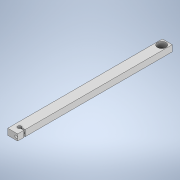
# Autodesk Inventor part: Arm
Saved by Autodesk Inventor 2021.3 (Build 253353000, 353)
## iProperties
Created: 2021-10-18
Part Number: Arm
Material: Generisch
Document SubType Name: Modeling
Designer: bhelg
Density: 1 g/cm^3
Appearance: Vorgabe
Author: bhelg
Autodesk Inventor part; units mm, degrees
ref_plane "YZ Plane" through (0, 0, 0) normal (1, 0, 0) x (0, 1, 0)
ref_plane "XZ Plane" through (0, 0, 0) normal (0, 1, 0) x (-1, 0, 0)
ref_plane "XY Plane" through (0, 0, 0) normal (0, 0, 1) x (1, 0, 0)
sketch "Skizze2" plane through (0, 0, 0) normal (0, 1, 0) x (-1, 0, 0)
  line L0 (0, 0) -> (16, 0)
  line L1 (16, 0) -> (16, 250)
  line L2 (16, 250) -> (0, 250)
  line L3 (0, 250) -> (0, 0)
  dimension "d0" = 16
  dimension "d1" = 250
  constraints: 8 end point, 2 parallel, 1 horizontal, 1 perpendicular
  measures "d0" distance of L2.end L1.end
  measures "d1" distance of L1.end L0.end
extrude "Extrusion1" add sketch "Skizze2" along normal blind 10
sketch "Skizze3" plane through (0, 0, 250) normal (1, 0, 0) x (0, 0, -1)
  line L0 (250, 0) -> (0, 0) projected
  line L1 (250, 10) -> (0, 10) projected
  line L2 (10, 0) -> (12, 0)
  line L3 (12, 0) -> (12, 10)
  line L4 (12, 10) -> (10, 10)
  line L5 (10, 10) -> (10, 0)
  line L6 (0, 0) -> (0, 10) projected
  point P0 (10, 10)
  point P1 (12, 0)
  dimension "d4" = 2
  dimension "d5" = 10
  constraints: 8 end point, 2 parallel, 2 point on line, 1 horizontal, 1 perpendicular
  measures "d4" distance between parallel lines of L3 L5
  measures "d5" distance between parallel lines of L6 L5
extrude "Extrusion2" cut sketch "Skizze3" against normal blind 7.5 contours L0 L5 L1 L3
sketch "Skizze4" plane through (-16, 0, 250) normal (0, 0, 1) x (1, 0, 0)
  line L0 (0, 0) -> (16, 0) projected
  line L1 (16, 0) -> (16, 10) projected
  point P0 (13.5, 5)
  dimension "d8" = 5
  dimension "d9" = 2.5
  measures "d8" distance from line of point (13.5, 5) L0
  measures "d9" distance from line of L1 point (13.5, 5)
hole "Bohrung1" at (-2.5, 5, 250) direction (0, 0, -1) diameter 4.2 depth 12
sketch "Skizze5" plane through (0, 10, 0) normal (0, 1, 0) x (1, 0, 0)
  line L0 (-16, -250) -> (0, -250) projected
  line L1 (-16, 0) -> (-16, -250) projected
  point P0 (0, 0)
  point P1 (-8, -239)
  dimension "d17" = 11
  dimension "d18" = 8
  measures "d17" distance from line of point (-8, -239) L0
  measures "d18" distance from line of L1 point (-8, -239)
hole "Bohrung2" at (-8, 10, 239) direction (0, -1, 0) diameter 6 depth 18 tip angle 118
sketch "Skizze7" plane through (0, 10, 0) normal (0, 1, 0) x (1, 0, 0)
  circle A0 centre (-8, -9) radius 7.05
  line L0 (0, -238) -> (0, 0) projected
  line L1 (0, 0) -> (-16, 0) projected
  arc A1 (-5.1716, -238) -> (-5.1716, -240) centre (-8, -239) ccw projected
  dimension "d35" = 14.1
  dimension "d36" = 8
  dimension "d43" = 230
  constraints: 1 centre point
  measures "d35" diameter of A0
  measures "d36" distance from line of A0.centre L0
  measures "d43" distance of A0.centre A1.centre
extrude "Extrusion3" cut sketch "Skizze7" against normal blind 9
sketch "Skizze9" plane through (0, 10, 0) normal (0, 1, 0) x (1, 0, 0)
  circle A0 centre (-8, -9) radius 7.05 projected
  circle A1 centre (-8, -9) radius 6.05
  point P0 (0, 0)
  dimension "d40" = 12.1
  constraints: 1 centre point, 1 coincident
  measures "d40" diameter of A1
extrude "Extrusion4" cut sketch "Skizze9" against normal through all contours A1
sketch "Skizze10" plane through (-16, 0, 250) normal (0, 0, 1) x (1, 0, 0)
  circle A0 centre (13.5, 5) radius 2.1 projected
  point P0 (16, 0)
  constraints: 1 coincident
hole "Bohrung4" at (-2.5, 5, 250) direction (0, 0, -1) diameter 3.242 depth 18 tip angle 118 thread size "M4x0.7" class "6H" standard "ISO Metric profile"
